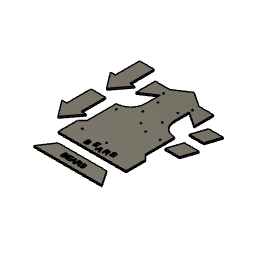
likhon bears final 3d (Autodesk Fusion 360 design; units mm, degrees)
Autodesk Fusion 360 part; units mm, degrees
note: some values were not read from the file. Chosen so that the rebuilt part matches the saved one: which bodies a step acts on.
(part 1 of 2)
sketch "Sketch1" plane through (0, 0, 0) normal (0, 1, 0) x (1, 0, 0)
  line L0 (-82.221, 0) -> (-82.221, -50)
  spline S0 degree 2 poles (7.3414, -90.0517) (7.4957, -89.8408) (7.4965, -89.6089) knots 0 0 0 1 1 1
  spline S1 degree 2 poles (7.4965, -89.6089) (7.4975, -89.3361) (7.2763, -89.1988) knots 0 0 0 1 1 1
  line L1 (-122.221, -50) -> (-112.221, -50)
  line L2 (-72.221, -50) -> (-97.221, -83.0105)
  line L3 (1.7193, -143.9734) -> (1.2998, -143.9755)
  spline S2 degree 2 poles (-7.3947, -90.6256) (-7.0097, -90.7327) (-6.7941, -91.0047) knots 0 0 0 1 1 1
  line L4 (-82.221, -50) -> (-72.221, -50)
  line L5 (1.7256, -141.8792) -> (1.4528, -143.2244)
  line L6 (-97.221, -83.0105) -> (-122.221, -50)
  line L7 (-0.1527, -146.0533) -> (0.8687, -141.048)
  spline S3 degree 2 poles (5.9982, -144.3505) (6.0211, -144.8176) (6.1618, -144.9806) knots 0 0 0 1 1 1
  spline S4 degree 2 poles (3.0979, -143.117) (3.3686, -143.0167) (3.521, -142.8045) knots 0 0 0 1 1 1
  spline S5 degree 2 poles (3.4484, -141.9522) (3.3115, -141.871) (2.8579, -141.8734) knots 0 0 0 1 1 1
  spline S6 degree 2 poles (6.1966, -143.4678) (5.928, -143.3003) (5.7732, -143.0317) knots 0 0 0 1 1 1
  line L8 (-3.5767, -144.1336) -> (-2.0794, -144.1259)
  spline S7 degree 2 poles (3.1685, -143.9114) (3.3673, -144.0877) (3.5427, -144.3767) knots 0 0 0 1 1 1
  spline S8 degree 2 poles (10.4231, -89.5514) (10.4223, -89.7662) (10.5889, -89.9067) knots 0 0 0 1 1 1
  spline S9 degree 2 poles (11.8704, -89.219) (11.6494, -89.0272) (11.2163, -89.0256) knots 0 0 0 1 1 1
  line L9 (2.8579, -141.8734) -> (1.7256, -141.8792)
  line L10 (1.2998, -143.9755) -> (0.8773, -146.048)
  line L11 (-112.221, -50) -> (-112.221, 0)
  spline S10 degree 2 poles (3.521, -142.8045) (3.6734, -142.5923) (3.6722, -142.3603) knots 0 0 0 1 1 1
  spline S11 degree 2 poles (10.6069, -89.1734) (10.4239, -89.3228) (10.4231, -89.5514) knots 0 0 0 1 1 1
  line L12 (0.8687, -141.048) -> (3.089, -141.0366)
  spline S12 degree 2 poles (4.4986, -141.5784) (4.6964, -141.8912) (4.6987, -142.338) knots 0 0 0 1 1 1
  line L13 (4.3186, -146.0303) -> (3.2135, -146.036)
  line L14 (-2.0794, -144.1259) -> (-2.3797, -142.1152)
  spline S13 degree 2 poles (2.2314, -144.0697) (2.0842, -143.9715) (1.7193, -143.9734) knots 0 0 0 1 1 1
  spline S14 degree 2 poles (7.7243, -145.0578) (7.9484, -144.8759) (7.9471, -144.6201) knots 0 0 0 1 1 1
  line L15 (5.0197, -144.4066) -> (5.9982, -144.3505)
  spline S15 degree 2 poles (4.6987, -142.338) (4.7019, -142.9758) (4.3221, -143.3921) knots 0 0 0 1 1 1
  spline S16 degree 2 poles (4.3221, -143.3921) (3.9422, -143.8085) (3.1685, -143.9114) knots 0 0 0 1 1 1
  line L16 (-9.4738, -90.2394) -> (-8.6894, -90.2423)
  circle A0 centre (20, -50) radius 1.5
  spline S17 degree 2 poles (-7.4625, -89.5612) (-7.4618, -89.3702) (-7.5705, -89.247) knots 0 0 0 1 1 1
  spline S18 degree 2 poles (6.9157, -90.3605) (7.1872, -90.2626) (7.3414, -90.0517) knots 0 0 0 1 1 1
  circle A1 centre (-19.4752, 45.0876) radius 1.5
  spline S19 degree 2 poles (3.2135, -146.036) (3.0784, -145.6138) (2.6849, -144.7188) knots 0 0 0 1 1 1
  spline S20 degree 2 poles (3.6722, -142.3603) (3.6708, -142.0875) (3.4484, -141.9522) knots 0 0 0 1 1 1
  spline S21 degree 2 poles (6.0681, -141.3521) (6.523, -140.9337) (7.3893, -140.9292) knots 0 0 0 1 1 1
  spline S22 degree 2 poles (-8.3614, -88.2244) (-7.8055, -88.2264) (-7.5839, -88.2613) knots 0 0 0 1 1 1
  spline S23 degree 2 poles (1.9985, -143.2216) (2.8273, -143.2173) (3.0979, -143.117) knots 0 0 0 1 1 1
  spline S24 degree 2 poles (2.6849, -144.7188) (2.471, -144.2356) (2.2314, -144.0697) knots 0 0 0 1 1 1
  spline S25 degree 2 poles (-10.4957, -143.0419) (-10.7261, -143.3484) (-11.2096, -143.5077) knots 0 0 0 1 1 1
  spline S26 degree 2 poles (-7.5468, -93.05) (-7.9977, -93.2257) (-8.7787, -93.2229) knots 0 0 0 1 1 1
  spline S27 degree 2 poles (-7.5798, -89.9257) (-7.4632, -89.7556) (-7.4625, -89.5612) knots 0 0 0 1 1 1
  line L17 (-112.221, 0) -> (-82.221, 0)
  spline S28 degree 2 poles (3.5427, -144.3767) (3.8902, -144.9616) (4.3186, -146.0303) knots 0 0 0 1 1 1
  spline S29 degree 2 poles (-8.6894, -90.2423) (-8.1607, -90.2442) (-7.9285, -90.17) knots 0 0 0 1 1 1
  spline S30 degree 2 poles (-6.5732, -88.8789) (-6.4411, -89.1352) (-6.4423, -89.4456) knots 0 0 0 1 1 1
  line L18 (-2.3797, -142.1152) -> (-3.5767, -144.1336)
  line L19 (1.4528, -143.2244) -> (1.9985, -143.2216)
  circle A2 centre (0, -10) radius 1.5
  spline S31 degree 2 poles (5.6165, -142.4015) (5.6132, -141.7705) (6.0681, -141.3521) knots 0 0 0 1 1 1
  spline S32 degree 2 poles (6.5981, -142.2771) (6.5992, -142.492) (6.767, -142.6309) knots 0 0 0 1 1 1
  spline S33 degree 2 poles (6.7786, -141.8976) (6.5969, -142.0486) (6.5981, -142.2771) knots 0 0 0 1 1 1
  line L20 (9.2899, -142.4304) -> (8.3045, -142.4798)
  line L21 (-11.1354, -93.2143) -> (-10.0702, -88.2182)
  spline S34 degree 2 poles (8.0425, -141.932) (7.8198, -141.7422) (7.3866, -141.7444) knots 0 0 0 1 1 1
  spline S35 degree 2 poles (8.4485, -145.6254) (7.9274, -146.097) (6.9929, -146.1018) knots 0 0 0 1 1 1
  spline S36 degree 2 poles (7.9471, -144.6201) (7.946, -144.3984) (7.761, -144.2459) knots 0 0 0 1 1 1
  spline S37 degree 2 poles (8.7539, -141.3349) (9.2387, -141.7451) (9.2899, -142.4304) knots 0 0 0 1 1 1
  spline S38 degree 2 poles (8.6105, -143.6174) (8.9635, -143.9566) (8.9663, -144.4921) knots 0 0 0 1 1 1
  spline S39 degree 2 poles (-11.3974, -142.1308) (-11.5072, -142.0086) (-11.7086, -141.9687) knots 0 0 0 1 1 1
  spline S40 degree 2 poles (-10.7944, -141.3466) (-10.5378, -141.4988) (-10.4034, -141.7539) knots 0 0 0 1 1 1
  spline S41 degree 2 poles (-11.4195, -141.1452) (-11.0509, -141.1945) (-10.7944, -141.3466) knots 0 0 0 1 1 1
  spline S42 degree 2 poles (-10.4034, -141.7539) (-10.2691, -142.009) (-10.2675, -142.3194) knots 0 0 0 1 1 1
  spline S43 degree 2 poles (7.3893, -140.9292) (8.2692, -140.9247) (8.7539, -141.3349) knots 0 0 0 1 1 1
  spline S44 degree 2 poles (7.3866, -141.7444) (6.9603, -141.7466) (6.7786, -141.8976) knots 0 0 0 1 1 1
  spline S45 degree 2 poles (8.9663, -144.4921) (8.9697, -145.1538) (8.4485, -145.6254) knots 0 0 0 1 1 1
  spline S46 degree 2 poles (6.0408, -91.3055) (5.8945, -91.2061) (5.5296, -91.2047) knots 0 0 0 1 1 1
  spline S47 degree 2 poles (6.4886, -91.9586) (6.2789, -91.4735) (6.0408, -91.3055) knots 0 0 0 1 1 1
  line L22 (-12.251, -141.951) -> (-13.0491, -141.9551)
  spline S48 degree 2 poles (7.048, -143.8846) (6.4652, -143.6352) (6.1966, -143.4678) knots 0 0 0 1 1 1
  spline S49 degree 2 poles (8.3045, -142.4798) (8.2651, -142.1219) (8.0425, -141.932) knots 0 0 0 1 1 1
  spline S50 degree 2 poles (6.767, -142.6309) (6.9349, -142.7733) (7.5092, -143.0193) knots 0 0 0 1 1 1
  spline S51 degree 2 poles (-6.9605, -88.4682) (-6.7053, -88.6226) (-6.5732, -88.8789) knots 0 0 0 1 1 1
  spline S52 degree 2 poles (6.9929, -146.1018) (6.3483, -146.1052) (5.8748, -145.891) knots 0 0 0 1 1 1
  line L23 (-10.0702, -88.2182) -> (-8.3614, -88.2244)
  spline S53 degree 2 poles (5.8748, -145.891) (5.4014, -145.6769) (5.205, -145.2925) knots 0 0 0 1 1 1
  spline S54 degree 2 poles (7.5092, -143.0193) (8.3739, -143.3867) (8.6105, -143.6174) knots 0 0 0 1 1 1
  spline S55 degree 2 poles (5.7732, -143.0317) (5.6183, -142.763) (5.6165, -142.4015) knots 0 0 0 1 1 1
  spline S56 degree 2 poles (6.9953, -145.2423) (7.5001, -145.2397) (7.7243, -145.0578) knots 0 0 0 1 1 1
  spline S57 degree 2 poles (6.1618, -144.9806) (6.3882, -145.2455) (6.9953, -145.2423) knots 0 0 0 1 1 1
  spline S58 degree 2 poles (7.761, -144.2459) (7.6308, -144.134) (7.048, -143.8846) knots 0 0 0 1 1 1
  spline S59 degree 2 poles (10.7943, -92.52) (11.299, -92.5218) (11.5248, -92.3419) knots 0 0 0 1 1 1
  line L24 (6.6866, -89.1148) -> (5.5543, -89.1107)
  spline S60 degree 2 poles (10.0112, -90.7385) (9.7441, -90.5687) (9.5916, -90.2987) knots 0 0 0 1 1 1
  spline S61 degree 2 poles (-12.5076, -143.1358) (-11.9789, -143.1331) (-11.7474, -143.0569) knots 0 0 0 1 1 1
  line L25 (-0.733, -93.2522) -> (-1.7903, -93.2484)
  spline S62 degree 2 poles (7.2763, -89.1988) (7.1402, -89.1165) (6.6866, -89.1148) knots 0 0 0 1 1 1
  spline S63 degree 2 poles (11.7515, -91.9061) (11.7523, -91.6844) (11.5687, -91.5303) knots 0 0 0 1 1 1
  spline S64 degree 2 poles (11.5248, -92.3419) (11.7506, -92.1619) (11.7515, -91.9061) knots 0 0 0 1 1 1
  line L26 (-1.8236, -90.2196) -> (-2.0006, -91.0545)
  line L27 (1.8528, -92.1566) -> (-0.1287, -92.1493)
  line L28 (-2.1791, -93.2469) -> (-6.0843, -93.2327)
  spline S65 degree 2 poles (12.1276, -89.769) (12.0914, -89.4108) (11.8704, -89.219) knots 0 0 0 1 1 1
  line L29 (-1.3151, -88.25) -> (-1.4921, -89.085)
  spline S66 degree 2 poles (-11.4008, -142.8095) (-11.2857, -142.6384) (-11.2867, -142.444) knots 0 0 0 1 1 1
  spline S67 degree 2 poles (8.1374, -90.6464) (7.7539, -91.0594) (6.9793, -91.1555) knots 0 0 0 1 1 1
  spline S68 degree 2 poles (7.0057, -93.2804) (6.8742, -92.857) (6.4886, -91.9586) knots 0 0 0 1 1 1
  spline S69 degree 2 poles (12.5871, -88.6281) (13.0682, -89.0426) (13.1135, -89.7283) knots 0 0 0 1 1 1
  line L30 (8.1107, -93.2844) -> (7.0057, -93.2804)
  line L31 (13.1135, -89.7283) -> (12.1276, -89.769)
  line L32 (4.7046, -88.272) -> (6.925, -88.2801)
  spline S70 degree 2 poles (-11.7086, -141.9687) (-11.8213, -141.9488) (-12.251, -141.951) knots 0 0 0 1 1 1
  spline S71 degree 2 poles (9.9012, -88.6217) (10.3598, -88.2073) (11.2261, -88.2105) knots 0 0 0 1 1 1
  line L33 (-13.7344, -145.3181) -> (-12.7419, -145.313)
  line L34 (-1.4921, -89.085) -> (-4.1694, -89.0753)
  line L35 (1.7297, -91.3239) -> (1.4471, -89.3106)
  spline S72 degree 2 poles (9.963, -92.2509) (10.1872, -92.5178) (10.7943, -92.52) knots 0 0 0 1 1 1
  spline S73 degree 2 poles (8.5232, -89.5956) (8.5209, -90.2334) (8.1374, -90.6464) knots 0 0 0 1 1 1
  spline S74 degree 2 poles (7.3493, -91.6241) (7.6917, -92.2119) (8.1107, -93.2844) knots 0 0 0 1 1 1
  spline S75 degree 2 poles (-10.2675, -142.3194) (-10.2654, -142.7355) (-10.4957, -143.0419) knots 0 0 0 1 1 1
  spline S76 degree 2 poles (-11.3404, -145.9334) (-11.7897, -146.1131) (-12.5707, -146.1171) knots 0 0 0 1 1 1
  line L36 (1.4471, -89.3106) -> (0.2324, -91.3185)
  spline S77 degree 2 poles (10.8589, -91.1628) (10.2783, -90.9083) (10.0112, -90.7385) knots 0 0 0 1 1 1
  line L37 (-4.4123, -90.2101) -> (-1.8236, -90.2196)
  spline S78 degree 2 poles (-11.2867, -142.444) (-11.2877, -142.253) (-11.3974, -142.1308) knots 0 0 0 1 1 1
  line L38 (5.5296, -91.2047) -> (5.1101, -91.2032)
  line L39 (-12.5707, -146.1171) -> (-14.9274, -146.1292)
  spline S79 degree 2 poles (-11.7474, -143.0569) (-11.5158, -142.9807) (-11.4008, -142.8095) knots 0 0 0 1 1 1
  line L40 (-4.1694, -89.0753) -> (-4.4123, -90.2101)
  line L41 (2.9914, -93.2658) -> (2.0159, -93.2622)
  line L42 (2.1978, -88.2628) -> (2.9914, -93.2658)
  line L43 (2.0159, -93.2622) -> (1.8528, -92.1566)
  line L44 (-13.292, -143.1399) -> (-12.5076, -143.1358)
  line L45 (8.826, -91.667) -> (9.805, -91.6194)
  spline S80 degree 2 poles (9.5916, -90.2987) (9.4391, -90.0287) (9.4404, -89.6671) knots 0 0 0 1 1 1
  line L46 (-0.1287, -92.1493) -> (-0.733, -93.2522)
  line L47 (1.0553, -88.2587) -> (2.1978, -88.2628)
  line L48 (0.2324, -91.3185) -> (1.7297, -91.3239)
  spline S81 degree 2 poles (8.3298, -88.8343) (8.5248, -89.1488) (8.5232, -89.5956) knots 0 0 0 1 1 1
  spline S82 degree 2 poles (11.2261, -88.2105) (12.106, -88.2137) (12.5871, -88.6281) knots 0 0 0 1 1 1
  spline S83 degree 2 poles (9.805, -91.6194) (9.8238, -92.0867) (9.963, -92.2509) knots 0 0 0 1 1 1
  line L49 (-2.0006, -91.0545) -> (-4.5893, -91.0451)
  line L50 (-4.5893, -91.0451) -> (-4.908, -92.4014)
  line L51 (5.1101, -91.2032) -> (4.6694, -93.2719)
  line L52 (-6.0843, -93.2327) -> (-5.0224, -88.2365)
  line L53 (5.5543, -89.1107) -> (5.2697, -90.4535)
  spline S84 degree 2 poles (9.4404, -89.6671) (9.4427, -89.0362) (9.9012, -88.6217) knots 0 0 0 1 1 1
  line L54 (-5.0224, -88.2365) -> (-1.3151, -88.25)
  line L55 (-1.9987, -92.412) -> (-2.1791, -93.2469)
  line L56 (-1.7903, -93.2484) -> (1.0553, -88.2587)
  line L57 (-13.0491, -141.9551) -> (-13.292, -143.1399)
  spline S85 degree 2 poles (6.925, -88.2801) (7.4979, -88.2822) (7.8164, -88.401) knots 0 0 0 1 1 1
  spline S86 degree 2 poles (6.9793, -91.1555) (7.1765, -91.3335) (7.3493, -91.6241) knots 0 0 0 1 1 1
  spline S87 degree 2 poles (11.5687, -91.5303) (11.4395, -91.4173) (10.8589, -91.1628) knots 0 0 0 1 1 1
  line L58 (-4.908, -92.4014) -> (-1.9987, -92.412)
  line L59 (-9.6578, -91.1085) -> (-9.9354, -92.4138)
  spline S88 degree 2 poles (-11.6257, -144.163) (-11.8107, -144.002) (-12.2405, -144.0042) knots 0 0 0 1 1 1
  line L60 (-12.2405, -144.0042) -> (-13.4683, -144.0105)
  spline S89 degree 2 poles (-7.8166, -91.2772) (-8.0002, -91.1145) (-8.4299, -91.113) knots 0 0 0 1 1 1
  line L61 (80, 0) -> (110, 0)
  line L62 (5.2697, -90.4535) -> (5.8154, -90.4554)
  spline S90 degree 2 poles (-7.9285, -90.17) (-7.6963, -90.0958) (-7.5798, -89.9257) knots 0 0 0 1 1 1
  line L63 (70, 20) -> (80, 50)
  line L64 (-1.949, -144.9575) -> (-3.9305, -144.9676)
  line L65 (-5.5824, -146.0812) -> (-2.7807, -141.0667)
  line L66 (70, -30) -> (80, 0)
  line L67 (-13.4683, -144.0105) -> (-13.7344, -145.3181)
  circle A3 centre (-50, -10) radius 1.5
  circle A4 centre (20.1369, 46.1679) radius 1.5
  circle A5 centre (20.8571, 13.7581) radius 1.5
  spline S91 degree 2 poles (9.6681, -93.1588) (9.1965, -92.9405) (9.0035, -92.5544) knots 0 0 0 1 1 1
  spline S92 degree 2 poles (3.089, -141.0366) (3.6619, -141.0336) (3.9814, -141.1497) knots 0 0 0 1 1 1
  spline S93 degree 2 poles (-11.9051, -145.2286) (-11.6923, -145.1474) (-11.5654, -144.9625) knots 0 0 0 1 1 1
  spline S94 degree 2 poles (-11.4395, -144.5731) (-11.4407, -144.3241) (-11.6257, -144.163) knots 0 0 0 1 1 1
  circle A6 centre (-50, -80) radius 1.5
  spline S95 degree 2 poles (11.3276, -90.3016) (12.1891, -90.6765) (12.4236, -90.9093) knots 0 0 0 1 1 1
  line L68 (-7.998, -141.9291) -> (-8.2309, -143.0661)
  spline S96 degree 2 poles (-8.9429, -92.4174) (-8.3187, -92.4196) (-8.1053, -92.3403) knots 0 0 0 1 1 1
  spline S97 degree 2 poles (-12.7419, -145.313) (-12.1178, -145.3098) (-11.9051, -145.2286) knots 0 0 0 1 1 1
  line L69 (3.6394, -93.2681) -> (4.7046, -88.272)
  spline S98 degree 2 poles (10.5889, -89.9067) (10.7555, -90.0505) (11.3276, -90.3016) knots 0 0 0 1 1 1
  line L70 (-3.9305, -144.9676) -> (-4.5251, -146.0758)
  circle A7 centre (29.8599, 66.6942) radius 1.5
  spline S99 degree 2 poles (-7.5839, -88.2613) (-7.2158, -88.3138) (-6.9605, -88.4682) knots 0 0 0 1 1 1
  spline S100 degree 2 poles (-11.2096, -143.5077) (-10.8236, -143.6115) (-10.6057, -143.8815) knots 0 0 0 1 1 1
  line L71 (110, 0) -> (100, -30)
  spline S101 degree 2 poles (-7.8802, -89.0822) (-7.9927, -89.0613) (-8.4225, -89.0598) knots 0 0 0 1 1 1
  spline S102 degree 2 poles (9.0035, -92.5544) (8.8105, -92.1683) (8.826, -91.667) knots 0 0 0 1 1 1
  spline S103 degree 2 poles (-6.7941, -91.0047) (-6.5785, -91.2766) (-6.5798, -91.6177) knots 0 0 0 1 1 1
  spline S104 degree 2 poles (-10.6057, -143.8815) (-10.3877, -144.1516) (-10.386, -144.4926) knots 0 0 0 1 1 1
  line L72 (-8.7787, -93.2229) -> (-11.1354, -93.2143)
  line L73 (-1.7762, -146.0616) -> (-1.949, -144.9575)
  line L74 (100, -30) -> (70, -30)
  line L75 (-8.4225, -89.0598) -> (-9.2205, -89.0569)
  line L76 (-9.9354, -92.4138) -> (-8.9429, -92.4174)
  line L77 (-2.7807, -141.0667) -> (-1.6381, -141.0609)
  spline S105 degree 2 poles (-7.5705, -89.247) (-7.6792, -89.1239) (-7.8802, -89.0822) knots 0 0 0 1 1 1
  line L78 (-4.5251, -146.0758) -> (-5.5824, -146.0812)
  spline S106 degree 2 poles (5.8154, -90.4554) (6.6442, -90.4585) (6.9157, -90.3605) knots 0 0 0 1 1 1
  spline S107 degree 2 poles (10.7843, -93.3794) (10.1397, -93.3771) (9.6681, -93.1588) knots 0 0 0 1 1 1
  line L79 (0.8773, -146.048) -> (-0.1527, -146.0533)
  circle A8 centre (-30, 66.3341) radius 1.5
  line L80 (-8.4299, -91.113) -> (-9.6578, -91.1085)
  line L81 (-9.2205, -89.0569) -> (-9.4738, -90.2394)
  line L82 (4.6694, -93.2719) -> (3.6394, -93.2681)
  circle A9 centre (0, -80) radius 1.5
  spline S108 degree 2 poles (7.8164, -88.401) (8.1349, -88.5198) (8.3298, -88.8343) knots 0 0 0 1 1 1
  spline S109 degree 2 poles (12.2441, -92.9158) (11.7188, -93.3828) (10.7843, -93.3794) knots 0 0 0 1 1 1
  spline S110 degree 2 poles (11.2163, -89.0256) (10.7899, -89.024) (10.6069, -89.1734) knots 0 0 0 1 1 1
  line L83 (-1.6381, -141.0609) -> (-0.8007, -146.0566)
  spline S111 degree 2 poles (-7.6339, -91.6889) (-7.633, -91.4399) (-7.8166, -91.2772) knots 0 0 0 1 1 1
  line L84 (100, 20) -> (70, 20)
  line L85 (-0.8007, -146.0566) -> (-1.7762, -146.0616)
  line L86 (80, 50) -> (110, 50)
  spline S112 degree 2 poles (3.9814, -141.1497) (4.3009, -141.2657) (4.4986, -141.5784) knots 0 0 0 1 1 1
  spline S113 degree 2 poles (-8.1053, -92.3403) (-7.8918, -92.2609) (-7.7633, -92.0772) knots 0 0 0 1 1 1
  spline S114 degree 2 poles (-6.8387, -92.4711) (-7.096, -92.8743) (-7.5468, -93.05) knots 0 0 0 1 1 1
  line L87 (110, 50) -> (100, 20)
  spline S115 degree 2 poles (-7.7633, -92.0772) (-7.6347, -91.8935) (-7.6339, -91.6889) knots 0 0 0 1 1 1
  line L88 (60, 80) -> (60, 60)
  arc A10 (30, 30) -> (60, 0) centre (60, 30) ccw
  line L89 (30, 60) -> (30, 30)
  line L90 (-8.7074, -145.2616) -> (-5.7981, -145.2467)
  line L91 (30, 80) -> (60, 80)
  circle A11 centre (50, -50) radius 1.5
  line L92 (-14.9274, -146.1292) -> (-13.906, -141.1239)
  line L93 (-122.221, 50) -> (-97.221, 16.9895)
  line L94 (-50, -130) -> (50, -130)
  line L95 (-13.906, -141.1239) -> (-12.1973, -141.1151)
  line L96 (-60, 60) -> (-60, 80)
  line L97 (-8.2309, -143.0661) -> (-5.6423, -143.0528)
  line L98 (70, -70) -> (70, -110)
  line L99 (-50, -160) -> (-70, -160)
  spline S116 degree 2 poles (-12.1973, -141.1151) (-11.6414, -141.1122) (-11.4195, -141.1452) knots 0 0 0 1 1 1
  line L100 (-30, 60) -> (-60, 40)
  line L101 (70, -160) -> (50, -160)
  line L102 (-112.221, 50) -> (-122.221, 50)
  line L103 (-60, 40) -> (-60, 60)
  spline S117 degree 2 poles (5.205, -145.2925) (5.0086, -144.9081) (5.0197, -144.4066) knots 0 0 0 1 1 1
  line L104 (50, -130) -> (70, -160)
  spline S118 degree 2 poles (-10.386, -144.4926) (-10.3837, -144.9428) (-10.6374, -145.3483) knots 0 0 0 1 1 1
  line L105 (-5.7981, -145.2467) -> (-5.9712, -146.0832)
  spline S119 degree 2 poles (-10.6374, -145.3483) (-10.8911, -145.7537) (-11.3404, -145.9334) knots 0 0 0 1 1 1
  line L106 (-5.3207, -141.9154) -> (-7.998, -141.9291)
  line L107 (-70, -110) -> (-70, -70)
  line L108 (-8.8584, -141.098) -> (-5.151, -141.0789)
  line L109 (-60, 80) -> (-30, 80)
  line L110 (-30, 80) -> (0, 100)
  line L111 (-70, -70) -> (-60, -60)
  line L112 (-5.6423, -143.0528) -> (-5.8119, -143.8893)
  line L113 (-9.8763, -146.1032) -> (-8.8584, -141.098)
  line L114 (70, -110) -> (60, -110)
  line L115 (-5.151, -141.0789) -> (-5.3207, -141.9154)
  spline S120 degree 2 poles (12.7717, -91.7871) (12.7693, -92.4487) (12.2441, -92.9158) knots 0 0 0 1 1 1
  spline S121 degree 2 poles (12.4236, -90.9093) (12.7737, -91.2516) (12.7717, -91.7871) knots 0 0 0 1 1 1
  line L116 (0, 100) -> (30, 80)
  line L117 (-72.221, 50) -> (-82.221, 50)
  line L118 (60, -110) -> (-60, -110)
  line L119 (-112.221, 100) -> (-112.221, 50)
  line L120 (60, 60) -> (60, 40)
  line L121 (-97.221, 16.9895) -> (-72.221, 50)
  line L122 (-60, -60) -> (-60, 0)
  line L123 (-82.221, 100) -> (-112.221, 100)
  line L124 (50, -160) -> (-50, -160)
  spline S122 degree 2 poles (-6.4423, -89.4456) (-6.4438, -89.8617) (-6.6768, -90.1661) knots 0 0 0 1 1 1
  spline S123 degree 2 poles (-11.5654, -144.9625) (-11.4384, -144.7777) (-11.4395, -144.5731) knots 0 0 0 1 1 1
  spline S124 degree 2 poles (-6.6768, -90.1661) (-6.9098, -90.4705) (-7.3947, -90.6256) knots 0 0 0 1 1 1
  line L125 (-60, -110) -> (-70, -110)
  line L126 (60, -60) -> (70, -70)
  circle A12 centre (20, -20) radius 1.5
  line L127 (60, 0) -> (60, -60)
  line L128 (-82.221, 50) -> (-82.221, 100)
  line L129 (60, 40) -> (30, 60)
  circle A13 centre (-18.755, 13.3979) radius 1.5
  circle A14 centre (50, -20) radius 1.5
  line L130 (-8.4006, -143.9026) -> (-8.7074, -145.2616)
  arc A15 (-60, 0) -> (-30, 30) centre (-60, 30) ccw
  spline S125 degree 2 poles (-6.5798, -91.6177) (-6.5814, -92.0679) (-6.8387, -92.4711) knots 0 0 0 1 1 1
  line L131 (-5.8119, -143.8893) -> (-8.4006, -143.9026)
  line L132 (-5.9712, -146.0832) -> (-9.8763, -146.1032)
  line L133 (-70, -160) -> (-50, -130)
  line L134 (-30, 30) -> (-30, 60)
extrude "Extrude1" add sketch "Sketch1" along normal blind 3 contours L0 L1 L2 L4 L6 L11 L17 | S0 S1 S18 L24 S62 L53 L62 S106 | L3 L7 S7 L10 L12 S12 L13 S13 S15 S16 S19 S24 S28 S92 L79 S112 | S2 S22 S26 S30 L21 S51 L23 S99 S103 L72 S114 S122 S124 S125 | L5 S4 S5 L9 S10 S20 S23 L19 | S3 S6 S14 L15 S21 S31 S32 S33 L20 S34 S35 S36 S37 S38 S43 S44 S45 S48 S49 S50 S52 S53 S54 S55 S56 S57 S58 S117 | L8 L14 L18 | S8 S9 S11 S59 S60 S63 S64 S65 S69 L31 S71 S72 S77 L45 S80 S82 S83 S84 S87 S91 S95 S98 S102 S107 S109 S110 S120 S121 | L16 S17 S27 S29 S90 S101 L75 S105 L81 | A0 | S25 S40 S41 S42 S75 S76 L39 S100 S104 L92 L95 S116 S118 S119 | S39 L22 S61 S66 S70 S78 S79 L44 L57 | S46 S47 S67 S68 L30 L32 S73 S74 L38 S81 L51 S85 S86 L69 L82 S108 | L25 L27 L41 L42 L43 L46 L47 L56 | L26 L28 L29 L34 L37 L40 L49 L50 L52 L54 L55 L58 | L33 S88 L60 L67 S93 S94 S97 S123 | L35 L36 L48 | L59 S89 S96 L76 L80 S111 S113 S115 | L61 L66 L71 L74 | L63 L84 L86 L87 | L64 L65 L70 L73 L77 L78 L83 L85 | L68 L90 L97 L105 L106 L108 L112 L113 L115 L130 L131 L132 | L88 A10 L89 L91 L96 L98 L100 L103 L107 L109 L110 L111 L114 L116 L118 L120 L122 L125 L126 L127 L129 A15 L134 | A11 | L93 L102 L117 L119 L121 L123 L128 | L94 L99 L101 L104 L124 L133 makes body 1 at (83.3333, 0, -30) makes body 2 at (-92.221, 0, -66.6667) makes body 3 at (-20.4017, 0, 50) makes body 4 at (83.3333, 0, 20) makes body 5 at (-102.221, 0, 16.6667) makes body 6 at (16.6667, 0, 150)
sketch "Sketch2" plane through (0, 3, 0) normal (0, 1, 0) x (-1, 0, 0)
  circle A0 centre (0, 10) radius 1.5
  circle A1 centre (18.755, -13.3979) radius 1.5
  circle A2 centre (-50, 20) radius 1.5
  circle A3 centre (50, 10) radius 1.5
  circle A4 centre (19.4752, -45.0876) radius 1.5
  circle A5 centre (30, -66.3341) radius 1.5
  circle A6 centre (50, 80) radius 1.5
  circle A7 centre (-20, 20) radius 1.5
  circle A8 centre (-20.1369, -46.1679) radius 1.5
  circle A9 centre (-29.8599, -66.6942) radius 1.5
  circle A10 centre (0, 80) radius 1.5
  circle A11 centre (-20.8571, -13.7581) radius 1.5
  arc A12 (60, 0) -> (30, -30) centre (60, -30) ccw
  line L0 (60, 0) -> (60, 60)
  line L1 (60, 60) -> (70, 70)
  line L2 (70, 70) -> (70, 110)
  line L3 (70, 110) -> (-70, 110)
  line L4 (-70, 110) -> (-70, 70)
  line L5 (-70, 70) -> (-60, 60)
  line L6 (-60, 60) -> (-60, 0)
  arc A13 (-30, -30) -> (-60, 0) centre (-60, -30) ccw
  line L7 (-30, -30) -> (-30, -60)
  line L8 (-30, -60) -> (-60, -40)
  line L9 (-60, -40) -> (-60, -80)
  line L10 (-60, -80) -> (-30, -80)
  line L11 (-30, -80) -> (0, -100)
  line L12 (0, -100) -> (30, -80)
  line L13 (30, -80) -> (60, -80)
  line L14 (60, -80) -> (60, -40)
  line L15 (60, -40) -> (30, -60)
  line L16 (30, -60) -> (30, -30)
  line L17 (20, 98) -> (20, 88)
  line L18 (20, 88) -> (16.2483, 88)
  spline S0 degree 2 poles (16.2483, 88) (15.1023, 88) (14.41, 88.3035) knots 0 0 0 1 1 1
  spline S1 degree 2 poles (14.41, 88.3035) (13.7176, 88.6071) (13.3254, 89.2381) knots 0 0 0 1 1 1
  spline S2 degree 2 poles (13.3254, 89.2381) (12.9332, 89.869) (12.9332, 90.558) knots 0 0 0 1 1 1
  spline S3 degree 2 poles (12.9332, 90.558) (12.9332, 91.1992) (13.281, 91.7653) knots 0 0 0 1 1 1
  spline S4 degree 2 poles (13.281, 91.7653) (13.6289, 92.3315) (14.3315, 92.6794) knots 0 0 0 1 1 1
  spline S5 degree 2 poles (14.3315, 92.6794) (13.4243, 92.9454) (12.9366, 93.5866) knots 0 0 0 1 1 1
  spline S6 degree 2 poles (12.9366, 93.5866) (12.4488, 94.2278) (12.4488, 95.101) knots 0 0 0 1 1 1
  spline S7 degree 2 poles (12.4488, 95.101) (12.4488, 95.8035) (12.7456, 96.4072) knots 0 0 0 1 1 1
  spline S8 degree 2 poles (12.7456, 96.4072) (13.0423, 97.0109) (13.4789, 97.3383) knots 0 0 0 1 1 1
  spline S9 degree 2 poles (13.4789, 97.3383) (13.9154, 97.6658) (14.5737, 97.8329) knots 0 0 0 1 1 1
  spline S10 degree 2 poles (14.5737, 97.8329) (15.2319, 98) (16.1869, 98) knots 0 0 0 1 1 1
  line L19 (16.1869, 98) -> (20, 98)
  line L20 (18.6767, 92.2019) -> (16.5143, 92.2019)
  spline S11 degree 2 poles (16.5143, 92.2019) (15.6344, 92.2019) (15.2524, 92.0859) knots 0 0 0 1 1 1
  spline S12 degree 2 poles (15.2524, 92.0859) (14.7476, 91.9359) (14.4918, 91.588) knots 0 0 0 1 1 1
  spline S13 degree 2 poles (14.4918, 91.588) (14.236, 91.2401) (14.236, 90.7149) knots 0 0 0 1 1 1
  spline S14 degree 2 poles (14.236, 90.7149) (14.236, 90.2169) (14.4748, 89.8383) knots 0 0 0 1 1 1
  spline S15 degree 2 poles (14.4748, 89.8383) (14.7135, 89.4598) (15.1569, 89.3199) knots 0 0 0 1 1 1
  spline S16 degree 2 poles (15.1569, 89.3199) (15.6003, 89.1801) (16.678, 89.1801) knots 0 0 0 1 1 1
  line L21 (16.678, 89.1801) -> (18.6767, 89.1801)
  line L22 (18.6767, 89.1801) -> (18.6767, 92.2019)
  line L23 (18.6767, 96.8199) -> (16.1869, 96.8199)
  spline S17 degree 2 poles (16.1869, 96.8199) (15.5457, 96.8199) (15.2865, 96.7722) knots 0 0 0 1 1 1
  spline S18 degree 2 poles (15.2865, 96.7722) (14.8295, 96.6903) (14.5225, 96.4993) knots 0 0 0 1 1 1
  spline S19 degree 2 poles (14.5225, 96.4993) (14.2156, 96.3083) (14.0177, 95.9434) knots 0 0 0 1 1 1
  spline S20 degree 2 poles (14.0177, 95.9434) (13.8199, 95.5784) (13.8199, 95.101) knots 0 0 0 1 1 1
  spline S21 degree 2 poles (13.8199, 95.101) (13.8199, 94.5416) (14.1064, 94.1289) knots 0 0 0 1 1 1
  spline S22 degree 2 poles (14.1064, 94.1289) (14.3929, 93.7162) (14.9011, 93.5491) knots 0 0 0 1 1 1
  spline S23 degree 2 poles (14.9011, 93.5491) (15.4093, 93.382) (16.3643, 93.382) knots 0 0 0 1 1 1
  line L24 (16.3643, 93.382) -> (18.6767, 93.382)
  line L25 (18.6767, 93.382) -> (18.6767, 96.8199)
  line L26 (10.6003, 98) -> (10.6003, 88)
  line L27 (10.6003, 88) -> (3.3697, 88)
  line L28 (3.3697, 88) -> (3.3697, 89.1801)
  line L29 (3.3697, 89.1801) -> (9.2769, 89.1801)
  line L30 (9.2769, 89.1801) -> (9.2769, 92.2428)
  line L31 (9.2769, 92.2428) -> (3.7449, 92.2428)
  line L32 (3.7449, 92.2428) -> (3.7449, 93.4161)
  line L33 (3.7449, 93.4161) -> (9.2769, 93.4161)
  line L34 (9.2769, 93.4161) -> (9.2769, 96.8199)
  line L35 (9.2769, 96.8199) -> (3.1378, 96.8199)
  line L36 (3.1378, 96.8199) -> (3.1378, 98)
  line L37 (3.1378, 98) -> (10.6003, 98)
  line L38 (2.4079, 98) -> (-1.4325, 88)
  line L39 (-1.4325, 88) -> (-2.8581, 88)
  line L40 (-2.8581, 88) -> (-6.9509, 98)
  line L41 (-6.9509, 98) -> (-5.4434, 98)
  line L42 (-5.4434, 98) -> (-4.2769, 94.9714)
  line L43 (-4.2769, 94.9714) -> (-0.0955, 94.9714)
  line L44 (-0.0955, 94.9714) -> (1.0027, 98)
  line L45 (1.0027, 98) -> (2.4079, 98)
  line L46 (-0.4775, 93.8936) -> (-3.8677, 93.8936)
  line L47 (-3.8677, 93.8936) -> (-2.824, 91.1241)
  spline S24 degree 2 poles (-2.824, 91.1241) (-2.3465, 89.8622) (-2.1146, 89.0505) knots 0 0 0 1 1 1
  spline S25 degree 2 poles (-2.1146, 89.0505) (-1.9236, 90.0123) (-1.5757, 90.9604) knots 0 0 0 1 1 1
  line L48 (-1.5757, 90.9604) -> (-0.4775, 93.8936)
  line L49 (-8.0287, 98) -> (-8.0287, 88)
  line L50 (-8.0287, 88) -> (-12.4625, 88)
  spline S26 degree 2 poles (-12.4625, 88) (-13.7995, 88) (-14.4952, 88.2694) knots 0 0 0 1 1 1
  spline S27 degree 2 poles (-14.4952, 88.2694) (-15.191, 88.5389) (-15.6071, 89.221) knots 0 0 0 1 1 1
  spline S28 degree 2 poles (-15.6071, 89.221) (-16.0232, 89.9031) (-16.0232, 90.7285) knots 0 0 0 1 1 1
  spline S29 degree 2 poles (-16.0232, 90.7285) (-16.0232, 91.7926) (-15.3342, 92.5225) knots 0 0 0 1 1 1
  spline S30 degree 2 poles (-15.3342, 92.5225) (-14.6453, 93.2524) (-13.206, 93.4502) knots 0 0 0 1 1 1
  spline S31 degree 2 poles (-13.206, 93.4502) (-13.7312, 93.7026) (-14.0041, 93.9482) knots 0 0 0 1 1 1
  spline S32 degree 2 poles (-14.0041, 93.9482) (-14.5839, 94.4802) (-15.1023, 95.2783) knots 0 0 0 1 1 1
  line L51 (-15.1023, 95.2783) -> (-16.8417, 98)
  line L52 (-16.8417, 98) -> (-15.1774, 98)
  line L53 (-15.1774, 98) -> (-13.854, 95.9195)
  spline S33 degree 2 poles (-13.854, 95.9195) (-13.2742, 95.0191) (-12.899, 94.5416) knots 0 0 0 1 1 1
  spline S34 degree 2 poles (-12.899, 94.5416) (-12.5239, 94.0641) (-12.2271, 93.8731) knots 0 0 0 1 1 1
  spline S35 degree 2 poles (-12.2271, 93.8731) (-11.9304, 93.6821) (-11.6235, 93.6071) knots 0 0 0 1 1 1
  spline S36 degree 2 poles (-11.6235, 93.6071) (-11.3984, 93.5593) (-10.8868, 93.5593) knots 0 0 0 1 1 1
  line L54 (-10.8868, 93.5593) -> (-9.352, 93.5593)
  line L55 (-9.352, 93.5593) -> (-9.352, 98)
  line L56 (-9.352, 98) -> (-8.0287, 98)
  line L57 (-9.352, 92.4134) -> (-12.1965, 92.4134)
  spline S37 degree 2 poles (-12.1965, 92.4134) (-13.1037, 92.4134) (-13.6153, 92.2258) knots 0 0 0 1 1 1
  spline S38 degree 2 poles (-13.6153, 92.2258) (-14.1269, 92.0382) (-14.3929, 91.6255) knots 0 0 0 1 1 1
  spline S39 degree 2 poles (-14.3929, 91.6255) (-14.6589, 91.2128) (-14.6589, 90.7285) knots 0 0 0 1 1 1
  spline S40 degree 2 poles (-14.6589, 90.7285) (-14.6589, 90.0191) (-14.1439, 89.5621) knots 0 0 0 1 1 1
  spline S41 degree 2 poles (-14.1439, 89.5621) (-13.6289, 89.105) (-12.5171, 89.105) knots 0 0 0 1 1 1
  line L58 (-12.5171, 89.105) -> (-9.352, 89.105)
  line L59 (-9.352, 89.105) -> (-9.352, 92.4134)
  line L60 (-17.6467, 94.7872) -> (-18.895, 94.678)
  spline S42 degree 2 poles (-18.895, 94.678) (-18.9836, 95.4284) (-19.3076, 95.9093) knots 0 0 0 1 1 1
  spline S43 degree 2 poles (-19.3076, 95.9093) (-19.6317, 96.3902) (-20.3138, 96.6869) knots 0 0 0 1 1 1
  spline S44 degree 2 poles (-20.3138, 96.6869) (-20.9959, 96.9836) (-21.8486, 96.9836) knots 0 0 0 1 1 1
  spline S45 degree 2 poles (-21.8486, 96.9836) (-22.6057, 96.9836) (-23.1855, 96.7585) knots 0 0 0 1 1 1
  spline S46 degree 2 poles (-23.1855, 96.7585) (-23.7653, 96.5334) (-24.0484, 96.1412) knots 0 0 0 1 1 1
  spline S47 degree 2 poles (-24.0484, 96.1412) (-24.3315, 95.749) (-24.3315, 95.2851) knots 0 0 0 1 1 1
  spline S48 degree 2 poles (-24.3315, 95.2851) (-24.3315, 94.8145) (-24.0587, 94.4632) knots 0 0 0 1 1 1
  spline S49 degree 2 poles (-24.0587, 94.4632) (-23.7858, 94.1119) (-23.1583, 93.8731) knots 0 0 0 1 1 1
  spline S50 degree 2 poles (-23.1583, 93.8731) (-22.7558, 93.7162) (-21.3779, 93.3854) knots 0 0 0 1 1 1
  spline S51 degree 2 poles (-21.3779, 93.3854) (-20, 93.0546) (-19.4475, 92.7613) knots 0 0 0 1 1 1
  spline S52 degree 2 poles (-19.4475, 92.7613) (-18.7312, 92.3861) (-18.3799, 91.8302) knots 0 0 0 1 1 1
  spline S53 degree 2 poles (-18.3799, 91.8302) (-18.0287, 91.2742) (-18.0287, 90.5853) knots 0 0 0 1 1 1
  spline S54 degree 2 poles (-18.0287, 90.5853) (-18.0287, 89.8281) (-18.4584, 89.1699) knots 0 0 0 1 1 1
  spline S55 degree 2 poles (-18.4584, 89.1699) (-18.8881, 88.5116) (-19.7135, 88.1705) knots 0 0 0 1 1 1
  spline S56 degree 2 poles (-19.7135, 88.1705) (-20.5389, 87.8295) (-21.5484, 87.8295) knots 0 0 0 1 1 1
  spline S57 degree 2 poles (-21.5484, 87.8295) (-22.6603, 87.8295) (-23.5095, 88.1876) knots 0 0 0 1 1 1
  spline S58 degree 2 poles (-23.5095, 88.1876) (-24.3588, 88.5457) (-24.8158, 89.2415) knots 0 0 0 1 1 1
  spline S59 degree 2 poles (-24.8158, 89.2415) (-25.2729, 89.9372) (-25.307, 90.8172) knots 0 0 0 1 1 1
  line L61 (-25.307, 90.8172) -> (-24.0382, 90.9127)
  spline S60 degree 2 poles (-24.0382, 90.9127) (-23.9359, 89.9645) (-23.3458, 89.4802) knots 0 0 0 1 1 1
  spline S61 degree 2 poles (-23.3458, 89.4802) (-22.7558, 88.9959) (-21.603, 88.9959) knots 0 0 0 1 1 1
  spline S62 degree 2 poles (-21.603, 88.9959) (-20.4025, 88.9959) (-19.8533, 89.4359) knots 0 0 0 1 1 1
  spline S63 degree 2 poles (-19.8533, 89.4359) (-19.3042, 89.8759) (-19.3042, 90.4966) knots 0 0 0 1 1 1
  spline S64 degree 2 poles (-19.3042, 90.4966) (-19.3042, 91.0355) (-19.693, 91.3834) knots 0 0 0 1 1 1
  spline S65 degree 2 poles (-19.693, 91.3834) (-20.075, 91.7312) (-21.6883, 92.0962) knots 0 0 0 1 1 1
  spline S66 degree 2 poles (-21.6883, 92.0962) (-23.3015, 92.4611) (-23.9018, 92.734) knots 0 0 0 1 1 1
  spline S67 degree 2 poles (-23.9018, 92.734) (-24.7749, 93.1364) (-25.191, 93.7538) knots 0 0 0 1 1 1
  spline S68 degree 2 poles (-25.191, 93.7538) (-25.6071, 94.3711) (-25.6071, 95.176) knots 0 0 0 1 1 1
  spline S69 degree 2 poles (-25.6071, 95.176) (-25.6071, 95.9741) (-25.1501, 96.6801) knots 0 0 0 1 1 1
  spline S70 degree 2 poles (-25.1501, 96.6801) (-24.693, 97.3861) (-23.837, 97.7783) knots 0 0 0 1 1 1
  spline S71 degree 2 poles (-23.837, 97.7783) (-22.9809, 98.1705) (-21.91, 98.1705) knots 0 0 0 1 1 1
  spline S72 degree 2 poles (-21.91, 98.1705) (-20.5525, 98.1705) (-19.6351, 97.7749) knots 0 0 0 1 1 1
  spline S73 degree 2 poles (-19.6351, 97.7749) (-18.7176, 97.3793) (-18.1958, 96.5846) knots 0 0 0 1 1 1
  spline S74 degree 2 poles (-18.1958, 96.5846) (-17.6739, 95.7899) (-17.6467, 94.7872) knots 0 0 0 1 1 1
extrude "Extrude2" cut sketch "Sketch2" against normal blind 3 contours L26 L27 L28 L29 L30 L31 L32 L33 L34 L35 L36 L37 bodies 3
sketch "Sketch3" plane through (0, 3, 0) normal (0, 1, 0) x (-1, 0, 0)
  line L0 (9.2769, 96.8199) -> (3.1378, 96.8199)
  line L1 (3.1378, 96.8199) -> (3.1378, 98)
  line L2 (3.1378, 98) -> (10.6003, 98)
  line L3 (10.6003, 98) -> (10.6003, 88)
  line L4 (10.6003, 88) -> (3.3697, 88)
  line L5 (3.3697, 88) -> (3.3697, 89.1801)
  line L6 (3.3697, 89.1801) -> (9.2769, 89.1801)
  line L7 (9.2769, 89.1801) -> (9.2769, 92.2428)
  line L8 (9.2769, 92.2428) -> (3.7449, 92.2428)
  line L9 (3.7449, 92.2428) -> (3.7449, 93.4161)
  line L10 (3.7449, 93.4161) -> (9.2769, 93.4161)
  line L11 (9.2769, 93.4161) -> (9.2769, 96.8199)
  circle A0 centre (0, 10) radius 1.5
  circle A1 centre (18.755, -13.3979) radius 1.5
  circle A2 centre (-50, 20) radius 1.5
  circle A3 centre (50, 10) radius 1.5
  circle A4 centre (19.4752, -45.0876) radius 1.5
  circle A5 centre (30, -66.3341) radius 1.5
  circle A6 centre (50, 80) radius 1.5
  circle A7 centre (-20, 20) radius 1.5
  circle A8 centre (-20.1369, -46.1679) radius 1.5
  circle A9 centre (-29.8599, -66.6942) radius 1.5
  circle A10 centre (0, 80) radius 1.5
  circle A11 centre (-20.8571, -13.7581) radius 1.5
  arc A12 (60, 0) -> (30, -30) centre (60, -30) ccw
  line L12 (60, 0) -> (60, 60)
  line L13 (60, 60) -> (70, 70)
  line L14 (70, 70) -> (70, 110)
  line L15 (70, 110) -> (-70, 110)
  line L16 (-70, 110) -> (-70, 70)
  line L17 (-70, 70) -> (-60, 60)
  line L18 (-60, 60) -> (-60, 0)
  arc A13 (-30, -30) -> (-60, 0) centre (-60, -30) ccw
  line L19 (-30, -30) -> (-30, -60)
  line L20 (-30, -60) -> (-60, -40)
  line L21 (-60, -40) -> (-60, -80)
  line L22 (-60, -80) -> (-30, -80)
  line L23 (-30, -80) -> (0, -100)
  line L24 (0, -100) -> (30, -80)
  line L25 (30, -80) -> (60, -80)
  line L26 (60, -80) -> (60, -40)
  line L27 (60, -40) -> (30, -60)
  line L28 (30, -60) -> (30, -30)
  line L29 (24.6701, 103.0379) -> (24.3621, 93.0427)
  line L30 (24.3621, 93.0427) -> (20.6122, 93.1582)
  spline S0 degree 2 poles (20.6122, 93.1582) (19.4667, 93.1935) (18.784, 93.5182) knots 0 0 0 1 1 1
  spline S1 degree 2 poles (18.784, 93.5182) (18.1014, 93.843) (17.7288, 94.4857) knots 0 0 0 1 1 1
  spline S2 degree 2 poles (17.7288, 94.4857) (17.3562, 95.1285) (17.3774, 95.8171) knots 0 0 0 1 1 1
  spline S3 degree 2 poles (17.3774, 95.8171) (17.3971, 96.458) (17.7623, 97.0132) knots 0 0 0 1 1 1
  spline S4 degree 2 poles (17.7623, 97.0132) (18.1274, 97.5683) (18.8404, 97.8944) knots 0 0 0 1 1 1
  spline S5 degree 2 poles (18.8404, 97.8944) (17.9418, 98.1883) (17.4741, 98.8442) knots 0 0 0 1 1 1
  spline S6 degree 2 poles (17.4741, 98.8442) (17.0063, 99.5001) (17.0332, 100.3728) knots 0 0 0 1 1 1
  spline S7 degree 2 poles (17.0332, 100.3728) (17.0548, 101.0751) (17.37, 101.6693) knots 0 0 0 1 1 1
  spline S8 degree 2 poles (17.37, 101.6693) (17.6852, 102.2636) (18.1316, 102.5774) knots 0 0 0 1 1 1
  spline S9 degree 2 poles (18.1316, 102.5774) (18.5781, 102.8912) (19.2412, 103.038) knots 0 0 0 1 1 1
  spline S10 degree 2 poles (19.2412, 103.038) (19.9043, 103.1848) (20.8588, 103.1554) knots 0 0 0 1 1 1
  line L31 (20.8588, 103.1554) -> (24.6701, 103.0379)
  line L32 (23.1688, 97.2833) -> (21.0075, 97.3499)
  spline S11 degree 2 poles (21.0075, 97.3499) (20.1279, 97.377) (19.7426, 97.2729) knots 0 0 0 1 1 1
  spline S12 degree 2 poles (19.7426, 97.2729) (19.2334, 97.1384) (18.967, 96.7986) knots 0 0 0 1 1 1
  spline S13 degree 2 poles (18.967, 96.7986) (18.7006, 96.4588) (18.6845, 95.9338) knots 0 0 0 1 1 1
  spline S14 degree 2 poles (18.6845, 95.9338) (18.6691, 95.436) (18.8961, 95.0503) knots 0 0 0 1 1 1
  spline S15 degree 2 poles (18.8961, 95.0503) (19.1231, 94.6645) (19.5619, 94.5111) knots 0 0 0 1 1 1
  spline S16 degree 2 poles (19.5619, 94.5111) (20.0008, 94.3577) (21.078, 94.3245) knots 0 0 0 1 1 1
  line L33 (21.078, 94.3245) -> (23.0757, 94.2629)
  line L34 (23.0757, 94.2629) -> (23.1688, 97.2833)
  line L35 (23.311, 101.8992) -> (20.8224, 101.9758)
  spline S17 degree 2 poles (20.8224, 101.9758) (20.1815, 101.9956) (19.921, 101.9558) knots 0 0 0 1 1 1
  spline S18 degree 2 poles (19.921, 101.9558) (19.4617, 101.8881) (19.149, 101.7066) knots 0 0 0 1 1 1
  spline S19 degree 2 poles (19.149, 101.7066) (18.8363, 101.5252) (18.6273, 101.1665) knots 0 0 0 1 1 1
  spline S20 degree 2 poles (18.6273, 101.1665) (18.4183, 100.8078) (18.4036, 100.3306) knots 0 0 0 1 1 1
  spline S21 degree 2 poles (18.4036, 100.3306) (18.3864, 99.7715) (18.6601, 99.3502) knots 0 0 0 1 1 1
  spline S22 degree 2 poles (18.6601, 99.3502) (18.9337, 98.9289) (19.4365, 98.7462) knots 0 0 0 1 1 1
  spline S23 degree 2 poles (19.4365, 98.7462) (19.9393, 98.5635) (20.8938, 98.5341) knots 0 0 0 1 1 1
  line L36 (20.8938, 98.5341) -> (23.2051, 98.4629)
  line L37 (23.2051, 98.4629) -> (23.311, 101.8992)
extrude "Extrude3" cut sketch "Sketch3" against normal blind 3 contours L29 L30 S0 S1 S2 S3 S4 S5 S6 S7 S8 S9 S10 L31 bodies 3 makes body 7 at (-21.6758, 3, 100.803) makes body 8 at (-20.4017, 3, 50)
sketch "Sketch4" plane through (0, 3, 0) normal (0, 1, 0) x (-1, 0, 0)
  spline S0 degree 2 poles (18.1316, 102.5774) (18.5781, 102.8912) (19.2412, 103.038) knots 0 0 0 1 1 1
  spline S1 degree 2 poles (19.2412, 103.038) (19.9043, 103.1848) (20.8588, 103.1554) knots 0 0 0 1 1 1
  line L0 (20.8588, 103.1554) -> (24.6701, 103.0379)
  line L1 (24.6701, 103.0379) -> (24.3621, 93.0427)
  line L2 (24.3621, 93.0427) -> (20.6122, 93.1582)
  spline S2 degree 2 poles (20.6122, 93.1582) (19.4667, 93.1935) (18.784, 93.5182) knots 0 0 0 1 1 1
  spline S3 degree 2 poles (18.784, 93.5182) (18.1014, 93.843) (17.7288, 94.4857) knots 0 0 0 1 1 1
  spline S4 degree 2 poles (17.7288, 94.4857) (17.3562, 95.1285) (17.3774, 95.8171) knots 0 0 0 1 1 1
  spline S5 degree 2 poles (17.3774, 95.8171) (17.3971, 96.458) (17.7623, 97.0132) knots 0 0 0 1 1 1
  spline S6 degree 2 poles (17.7623, 97.0132) (18.1274, 97.5683) (18.8404, 97.8944) knots 0 0 0 1 1 1
  spline S7 degree 2 poles (18.8404, 97.8944) (17.9418, 98.1883) (17.4741, 98.8442) knots 0 0 0 1 1 1
  spline S8 degree 2 poles (17.4741, 98.8442) (17.0063, 99.5001) (17.0332, 100.3728) knots 0 0 0 1 1 1
  spline S9 degree 2 poles (17.0332, 100.3728) (17.0548, 101.0751) (17.37, 101.6693) knots 0 0 0 1 1 1
  spline S10 degree 2 poles (17.37, 101.6693) (17.6852, 102.2636) (18.1316, 102.5774) knots 0 0 0 1 1 1
  line L3 (9.2769, 96.8199) -> (3.1378, 96.8199)
  line L4 (3.1378, 96.8199) -> (3.1378, 98)
  line L5 (3.1378, 98) -> (10.6003, 98)
  line L6 (10.6003, 98) -> (10.6003, 88)
  line L7 (10.6003, 88) -> (3.3697, 88)
  line L8 (3.3697, 88) -> (3.3697, 89.1801)
  line L9 (3.3697, 89.1801) -> (9.2769, 89.1801)
  line L10 (9.2769, 89.1801) -> (9.2769, 92.2428)
  line L11 (9.2769, 92.2428) -> (3.7449, 92.2428)
  line L12 (3.7449, 92.2428) -> (3.7449, 93.4161)
  line L13 (3.7449, 93.4161) -> (9.2769, 93.4161)
  line L14 (9.2769, 93.4161) -> (9.2769, 96.8199)
  circle A0 centre (0, 10) radius 1.5
  circle A1 centre (18.755, -13.3979) radius 1.5
  circle A2 centre (-50, 20) radius 1.5
  circle A3 centre (50, 10) radius 1.5
  circle A4 centre (19.4752, -45.0876) radius 1.5
  circle A5 centre (30, -66.3341) radius 1.5
  circle A6 centre (50, 80) radius 1.5
  circle A7 centre (-20, 20) radius 1.5
  circle A8 centre (-20.1369, -46.1679) radius 1.5
  circle A9 centre (-29.8599, -66.6942) radius 1.5
  circle A10 centre (0, 80) radius 1.5
  circle A11 centre (-20.8571, -13.7581) radius 1.5
  arc A12 (60, 0) -> (30, -30) centre (60, -30) ccw
  line L15 (60, 0) -> (60, 60)
  line L16 (60, 60) -> (70, 70)
  line L17 (70, 70) -> (70, 110)
  line L18 (70, 110) -> (-70, 110)
  line L19 (-70, 110) -> (-70, 70)
  line L20 (-70, 70) -> (-60, 60)
  line L21 (-60, 60) -> (-60, 0)
  arc A13 (-30, -30) -> (-60, 0) centre (-60, -30) ccw
  line L22 (-30, -30) -> (-30, -60)
  line L23 (-30, -60) -> (-60, -40)
  line L24 (-60, -40) -> (-60, -80)
  line L25 (-60, -80) -> (-30, -80)
  line L26 (-30, -80) -> (0, -100)
  line L27 (0, -100) -> (30, -80)
  line L28 (30, -80) -> (60, -80)
  line L29 (60, -80) -> (60, -40)
  line L30 (60, -40) -> (30, -60)
  line L31 (30, -60) -> (30, -30)
  line L32 (0.6012, 103.5414) -> (-3.5606, 93.6708)
  line L33 (-3.5606, 93.6708) -> (-4.9855, 93.717)
  line L34 (-4.9855, 93.717) -> (-8.7527, 103.8441)
  line L35 (-8.7527, 103.8441) -> (-7.246, 103.7953)
  line L36 (-7.246, 103.7953) -> (-6.1781, 100.7305)
  line L37 (-6.1781, 100.7305) -> (-1.9988, 100.5953)
  line L38 (-1.9988, 100.5953) -> (-0.8032, 103.5868)
  line L39 (-0.8032, 103.5868) -> (0.6012, 103.5414)
  line L40 (-2.4155, 99.5305) -> (-5.8039, 99.6401)
  line L41 (-5.8039, 99.6401) -> (-4.8504, 96.8384)
  spline S11 degree 2 poles (-4.8504, 96.8384) (-4.4139, 95.5616) (-4.2084, 94.7428) knots 0 0 0 1 1 1
  spline S12 degree 2 poles (-4.2084, 94.7428) (-3.9864, 95.698) (-3.608, 96.6344) knots 0 0 0 1 1 1
  line L42 (-3.608, 96.6344) -> (-2.4155, 99.5305)
extrude "Extrude4" cut sketch "Sketch4" against normal blind 3 contours L32 L33 L34 L35 L36 L37 L38 L39 bodies 8 makes body 9 at (-20.4017, 3, 50)
sketch "Sketch5" plane through (0, 3, 0) normal (0, 1, 0) x (-1, 0, 0)
  arc A0 (60, 0) -> (30, -30) centre (60, -30) ccw
  line L0 (60, 0) -> (60, 60)
  line L1 (60, 60) -> (70, 70)
  line L2 (70, 70) -> (70, 110)
  line L3 (70, 110) -> (-70, 110)
  line L4 (-70, 110) -> (-70, 70)
  line L5 (-70, 70) -> (-60, 60)
  line L6 (-60, 60) -> (-60, 0)
  arc A1 (-30, -30) -> (-60, 0) centre (-60, -30) ccw
  line L7 (-30, -30) -> (-30, -60)
  line L8 (-30, -60) -> (-60, -40)
  line L9 (-60, -40) -> (-60, -80)
  line L10 (-60, -80) -> (-30, -80)
  line L11 (-30, -80) -> (0, -100)
  line L12 (0, -100) -> (30, -80)
  line L13 (30, -80) -> (60, -80)
  line L14 (60, -80) -> (60, -40)
  line L15 (60, -40) -> (30, -60)
  line L16 (30, -60) -> (30, -30)
  circle A2 centre (-20.8571, -13.7581) radius 1.5
  circle A3 centre (0, 80) radius 1.5
  circle A4 centre (-29.8599, -66.6942) radius 1.5
  circle A5 centre (-20.1369, -46.1679) radius 1.5
  circle A6 centre (-20, 20) radius 1.5
  circle A7 centre (50, 80) radius 1.5
  circle A8 centre (30, -66.3341) radius 1.5
  circle A9 centre (19.4752, -45.0876) radius 1.5
  circle A10 centre (50, 10) radius 1.5
  circle A11 centre (-50, 20) radius 1.5
  circle A12 centre (18.755, -13.3979) radius 1.5
  circle A13 centre (0, 10) radius 1.5
  line L17 (9.2769, 96.8199) -> (3.1378, 96.8199)
  line L18 (3.1378, 96.8199) -> (3.1378, 98)
  line L19 (3.1378, 98) -> (10.6003, 98)
  line L20 (10.6003, 98) -> (10.6003, 88)
  line L21 (10.6003, 88) -> (3.3697, 88)
  line L22 (3.3697, 88) -> (3.3697, 89.1801)
  line L23 (3.3697, 89.1801) -> (9.2769, 89.1801)
  line L24 (9.2769, 89.1801) -> (9.2769, 92.2428)
  line L25 (9.2769, 92.2428) -> (3.7449, 92.2428)
  line L26 (3.7449, 92.2428) -> (3.7449, 93.4161)
  line L27 (3.7449, 93.4161) -> (9.2769, 93.4161)
  line L28 (9.2769, 93.4161) -> (9.2769, 96.8199)
  spline S0 degree 2 poles (18.1316, 102.5774) (18.5781, 102.8912) (19.2412, 103.038) knots 0 0 0 1 1 1
  spline S1 degree 2 poles (19.2412, 103.038) (19.9043, 103.1848) (20.8588, 103.1554) knots 0 0 0 1 1 1
  line L29 (20.8588, 103.1554) -> (24.6701, 103.0379)
  line L30 (24.6701, 103.0379) -> (24.3621, 93.0427)
  line L31 (24.3621, 93.0427) -> (20.6122, 93.1582)
  spline S2 degree 2 poles (20.6122, 93.1582) (19.4667, 93.1935) (18.784, 93.5182) knots 0 0 0 1 1 1
  spline S3 degree 2 poles (18.784, 93.5182) (18.1014, 93.843) (17.7288, 94.4857) knots 0 0 0 1 1 1
  spline S4 degree 2 poles (17.7288, 94.4857) (17.3562, 95.1285) (17.3774, 95.8171) knots 0 0 0 1 1 1
  spline S5 degree 2 poles (17.3774, 95.8171) (17.3971, 96.458) (17.7623, 97.0132) knots 0 0 0 1 1 1
  spline S6 degree 2 poles (17.7623, 97.0132) (18.1274, 97.5683) (18.8404, 97.8944) knots 0 0 0 1 1 1
  spline S7 degree 2 poles (18.8404, 97.8944) (17.9418, 98.1883) (17.4741, 98.8442) knots 0 0 0 1 1 1
  spline S8 degree 2 poles (17.4741, 98.8442) (17.0063, 99.5001) (17.0332, 100.3728) knots 0 0 0 1 1 1
  spline S9 degree 2 poles (17.0332, 100.3728) (17.0548, 101.0751) (17.37, 101.6693) knots 0 0 0 1 1 1
  spline S10 degree 2 poles (17.37, 101.6693) (17.6852, 102.2636) (18.1316, 102.5774) knots 0 0 0 1 1 1
  line L32 (-6.1781, 100.7305) -> (-1.9988, 100.5953)
  line L33 (-1.9988, 100.5953) -> (-0.8032, 103.5868)
  line L34 (-0.8032, 103.5868) -> (0.6012, 103.5414)
  line L35 (0.6012, 103.5414) -> (-3.5606, 93.6708)
  line L36 (-3.5606, 93.6708) -> (-4.9855, 93.717)
  line L37 (-4.9855, 93.717) -> (-8.7527, 103.8441)
  line L38 (-8.7527, 103.8441) -> (-7.246, 103.7953)
  line L39 (-7.246, 103.7953) -> (-6.1781, 100.7305)
  line L40 (-12.4876, 101.6712) -> (-12.4876, 91.6712)
  line L41 (-12.4876, 91.6712) -> (-16.9215, 91.6712)
  spline S11 degree 2 poles (-16.9215, 91.6712) (-18.2585, 91.6712) (-18.9542, 91.9406) knots 0 0 0 1 1 1
  spline S12 degree 2 poles (-18.9542, 91.9406) (-19.65, 92.2101) (-20.0661, 92.8922) knots 0 0 0 1 1 1
  spline S13 degree 2 poles (-20.0661, 92.8922) (-20.4822, 93.5743) (-20.4822, 94.3997) knots 0 0 0 1 1 1
  spline S14 degree 2 poles (-20.4822, 94.3997) (-20.4822, 95.4638) (-19.7932, 96.1937) knots 0 0 0 1 1 1
  spline S15 degree 2 poles (-19.7932, 96.1937) (-19.1043, 96.9236) (-17.665, 97.1214) knots 0 0 0 1 1 1
  spline S16 degree 2 poles (-17.665, 97.1214) (-18.1902, 97.3738) (-18.4631, 97.6193) knots 0 0 0 1 1 1
  spline S17 degree 2 poles (-18.4631, 97.6193) (-19.0429, 98.1514) (-19.5613, 98.9495) knots 0 0 0 1 1 1
  line L42 (-19.5613, 98.9495) -> (-21.3007, 101.6712)
  line L43 (-21.3007, 101.6712) -> (-19.6364, 101.6712)
  line L44 (-19.6364, 101.6712) -> (-18.313, 99.5907)
  spline S18 degree 2 poles (-18.313, 99.5907) (-17.7332, 98.6903) (-17.358, 98.2128) knots 0 0 0 1 1 1
  spline S19 degree 2 poles (-17.358, 98.2128) (-16.9829, 97.7353) (-16.6861, 97.5443) knots 0 0 0 1 1 1
  spline S20 degree 2 poles (-16.6861, 97.5443) (-16.3894, 97.3533) (-16.0825, 97.2783) knots 0 0 0 1 1 1
  spline S21 degree 2 poles (-16.0825, 97.2783) (-15.8574, 97.2305) (-15.3458, 97.2305) knots 0 0 0 1 1 1
  line L45 (-15.3458, 97.2305) -> (-13.811, 97.2305)
  line L46 (-13.811, 97.2305) -> (-13.811, 101.6712)
  line L47 (-13.811, 101.6712) -> (-12.4876, 101.6712)
  line L48 (-13.811, 96.0846) -> (-16.6555, 96.0846)
  spline S22 degree 2 poles (-16.6555, 96.0846) (-17.5627, 96.0846) (-18.0743, 95.897) knots 0 0 0 1 1 1
  spline S23 degree 2 poles (-18.0743, 95.897) (-18.5859, 95.7094) (-18.8519, 95.2967) knots 0 0 0 1 1 1
  spline S24 degree 2 poles (-18.8519, 95.2967) (-19.1179, 94.884) (-19.1179, 94.3997) knots 0 0 0 1 1 1
  spline S25 degree 2 poles (-19.1179, 94.3997) (-19.1179, 93.6903) (-18.6029, 93.2333) knots 0 0 0 1 1 1
  spline S26 degree 2 poles (-18.6029, 93.2333) (-18.0879, 92.7762) (-16.9761, 92.7762) knots 0 0 0 1 1 1
  line L49 (-16.9761, 92.7762) -> (-13.811, 92.7762)
  line L50 (-13.811, 92.7762) -> (-13.811, 96.0846)
extrude "Extrude5" cut sketch "Sketch5" against normal blind 3 contours L40 L41 S11 S12 S13 S14 S15 S16 S17 L42 L43 L44 S18 S19 S20 S21 L45 L46 L47 bodies 9 makes body 10 at (-20.4017, 3, 50)